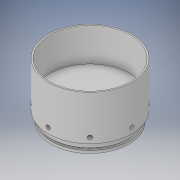
# Autodesk Inventor part: ForwardBulkHead
Saved by Autodesk Inventor 2017 (Build 210142000, 142)
## iProperties
Created: 2016-09-30
Part Number: ForwardBulkHead
Material: Generic
Document SubType Name: Modeling
Designer: cflannery
Density: 1 g/cm^3
Appearance: Default
Author: cflannery
Autodesk Inventor part; units mm, degrees
ref_plane "YZ Plane" through (0, 0, 0) normal (1, 0, 0) x (0, 1, 0)
ref_plane "XZ Plane" through (0, 0, 0) normal (0, 1, 0) x (-1, 0, 0)
ref_plane "XY Plane" through (0, 0, 0) normal (0, 0, 1) x (1, 0, 0)
sketch "Sketch1" plane through (0, 0, 0) normal (0, 0, 1) x (1, 0, 0)
  line L0 (0, 0) -> (-88.9, 0)
  line L1 (-88.9, 0) -> (-88.9, -12.7)
  line L2 (-88.9, -12.7) -> (-82.55, -12.7)
  line L3 (-82.55, -12.7) -> (-82.55, -17.4752)
  line L4 (-82.55, -17.4752) -> (-88.9, -17.4752)
  line L5 (-88.9, -17.4752) -> (-88.9, -23.8252)
  line L6 (-88.9, -23.8252) -> (0, -23.8252)
  line L7 (0, 0) -> (0, 146.0976) construction
  line L8 (-88.9, 0) -> (-95.25, 0)
  line L9 (-95.25, 0) -> (-95.25, 25.4)
  line L10 (-95.25, 25.4) -> (0, 25.4)
  line L11 (0, 25.4) -> (0, -23.8252)
  dimension "d1" = 4.7752
  dimension "d2" = 88.9
  dimension "d3" = 0
  dimension "d5" = 95.25
  dimension "d6" = 6.35
  dimension "d7" = 12.7
  dimension "d8" = 25.4
  dimension "d13" = 6.35
  dimension "d21" = 6.35
  constraints: 24 end point, 8 perpendicular, 2 horizontal, 2 vertical
  measures "d1" distance of L2.end L3.end
  measures "d2" distance from line of L7 L5.end
  measures "d3" distance between parallel lines of L7 L11
  measures "d5" distance between parallel lines of L7 L9
  measures "d6" distance of L4.end L5.end
  measures "d7" distance of L0.end L1.end
  measures "d8" distance of L8.end L9.end
  measures "d13" distance between parallel lines of L5 L3
  measures "d21" distance of L1.end L2.end
revolve "Revolution1" add sketch "Sketch1" angle 360 about axis through (0, 0, 0) along (0, 1, 0)
sketch "Sketch2" plane through (0, 25.4, 0) normal (0, 1, 0) x (1, 0, 0)
  circle A0 centre (0, 0) radius 95.25
  circle A1 centre (0, 0) radius 92.075
  dimension "d9" = 190.5
  dimension "d10" = 184.15
  constraints: 2 centre point, 2 coincident
  measures "d9" diameter of A0
  measures "d10" diameter of A1
extrude "Extrusion1" add sketch "Sketch2" along normal blind 76.2
sketch "Sketch3" plane through (0, 0, 0) normal (1, 0, 0) x (0, 1, 0)
  circle A0 centre (12.7, 0) radius 4.7625
  line L0 (0, -88.9) -> (0, 88.9) projected
  point P0 (0, 0)
  dimension "d14" = 12.7
  dimension "d15" = 9.525
  constraints: 1 centre point
  measures "d14" distance from line of L0 A0.centre
  measures "d15" diameter of A0
extrude "Extrusion2" cut sketch "Sketch3" against normal blind 127
pattern_circular "Circular Pattern1" count 8 over 360 about axis through (0, -10, 0) along (0, 1, 0) of "Extrusion2"
body "Solid1"
